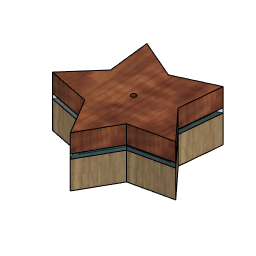
Star Prototype Non-Layered v3 (Autodesk Fusion 360 design; units mm, degrees)
Autodesk Fusion 360 part; units mm, degrees
note: some values were not read from the file. Set by a fixed rule: which face or edge a step refers to.
sketch "Sketch1" plane through (0, 0, 0) normal (0, 0, 1) x (1, 0, 0)
  line L0 (-201.2816, 81.9301) -> (-144.1352, 82.5743)
  line L1 (-144.1352, 82.5743) -> (-127.0887, 137.1228)
  line L2 (-127.0887, 137.1228) -> (-173.6998, 170.1914)
  line L3 (-173.6998, 170.1914) -> (-219.5535, 136.0805)
  line L4 (-219.5535, 136.0805) -> (-201.2816, 81.9301)
  line L5 (-196.6266, 153.136) -> (-226.1895, 192.8759) construction
  line L6 (-219.5535, 136.0805) -> (-226.1895, 192.8759)
  line L7 (-226.1895, 192.8759) -> (-173.6998, 170.1914)
  line L8 (-150.3942, 153.6571) -> (-121.7348, 194.0534) construction
  line L9 (-135.612, 109.8486) -> (-88.3366, 95.0749) construction
  line L10 (-172.7084, 82.2522) -> (-172.1501, 32.7254) construction
  line L11 (-210.4176, 109.0053) -> (-257.3479, 93.1697) construction
  line L12 (-173.6998, 170.1914) -> (-121.7348, 194.0534)
  line L13 (-127.0887, 137.1228) -> (-121.7348, 194.0534)
  line L14 (-127.0887, 137.1228) -> (-88.3366, 95.0749)
  line L15 (-144.1352, 82.5743) -> (-88.3366, 95.0749)
  line L16 (-144.1352, 82.5743) -> (-172.1501, 32.7254)
  line L17 (-257.3479, 93.1697) -> (-219.5535, 136.0805)
  circle A0 centre (-173.1518, 121.5798) radius 88.9 construction
  line L18 (-201.2816, 81.9301) -> (-257.3479, 93.1697)
  line L19 (-201.2816, 81.9301) -> (-172.1501, 32.7254)
  point P0 (-173.1518, 121.5798)
  dimension "d3" = 57.15
  dimension "d6" = 49.53
  dimension "d7" = 49.53
  dimension "d8" = 49.53
  dimension "d9" = 49.53
  dimension "d10" = 49.53
  dimension "d12" = 177.8
  constraint midpoint L3 L5.start
  constraint perpendicular L3 L5
  constraint midpoint L2 L8.start
  constraint perpendicular L2 L8
  constraint midpoint L1 L9.start
  constraint perpendicular L1 L9
  constraint midpoint L0 L10.start
  constraint perpendicular L0 L10
  constraint midpoint L4 L11.start
  constraint perpendicular L4 L11
  constraint coincident P0 A0.centre
  measures "d3" distance of L0.start L0.end
  measures "d6" distance of L5.start L5.end
  measures "d7" distance of L8.start L8.end
  measures "d8" distance of L9.start L9.end
  measures "d9" distance of L10.start L10.end
  measures "d10" distance of L11.start L11.end
  measures "d12" diameter of A0
extrude "Extrude1" add sketch "Sketch1" along normal blind 6.35 makes body 1
copy_body "CopyPasteBodies1" bodies 1 makes body 2
move_body "Move1" bodies 2 to x (1, 0, 0) y (0, 1, 0) z (0, 0, 1) at (0, 0, 6.35)
copy_body "CopyPasteBodies2" bodies 2 makes body 3
move_body "Move2" bodies 3 to x (1, 0, 0) y (0, 1, 0) z (0, 0, 1) at (0, 0, 6.35)
copy_body "CopyPasteBodies3" bodies 3 makes body 4
move_body "Move3" bodies 4 to x (1, 0, 0) y (0, 1, 0) z (0, 0, 1) at (0, 0, 6.35)
copy_body "CopyPasteBodies4" bodies 4 makes body 5
move_body "Move4" bodies 5 to x (1, 0, 0) y (0, 1, 0) z (0, 0, 1) at (0, 0, 6.35)
shell "Shell1" thickness 6.0325 removed faces 1 at (-163.5925, 118.5925, 31.75) on bodies 5
extrude "Extrude2" cut 1 faces at (-168.144, 128.6385, 31.4325) along direction (0, 0, -1) blind 6.0325 on bodies 5 bodies 5
copy_body "CopyPasteBodies6" bodies 5 makes body 6
move_body "Move5" bodies 6 to x (1, 0, 0) y (0, 1, 0) z (0, 0, 1) at (0, 0, 6.35)
copy_body "CopyPasteBodies7" bodies 6 makes body 7
move_body "Move6" bodies 7 to x (1, 0, 0) y (0, 1, 0) z (0, 0, 1) at (0, 0, 6.35)
copy_body "CopyPasteBodies8" bodies 1 2 3 4 makes body 8 makes body 9 makes body 10 makes body 11
move_body "Move7" bodies 8 9 10 11 to x (1, 0, 0) y (0, 1, 0) z (0, 0, 1) at (0, 0, 44.45)
sketch "Sketch2" plane through (0, 0, 69.85) normal (0, 0, 1) x (-1, 0, 0)
  line L0 (257.3479, -93.1697) -> (201.2816, -81.9301)
  line L1 (201.2816, -81.9301) -> (172.1501, -32.7254)
  line L2 (172.1501, -32.7254) -> (144.1352, -82.5743)
  line L3 (144.1352, -82.5743) -> (88.3366, -95.0749)
  line L4 (88.3366, -95.0749) -> (127.0887, -137.1228)
  line L5 (127.0887, -137.1228) -> (121.7348, -194.0534)
  line L6 (121.7348, -194.0534) -> (173.6998, -170.1914)
  line L7 (173.6998, -170.1914) -> (226.1895, -192.8759)
  line L8 (226.1895, -192.8759) -> (219.5535, -136.0805)
  line L9 (219.5535, -136.0805) -> (257.3479, -93.1697)
  line L10 (172.1501, -32.7254) -> (173.6998, -170.1914) construction
  line L11 (121.7348, -194.0534) -> (201.2816, -81.9301) construction
  line L12 (144.1352, -82.5743) -> (226.1895, -192.8759) construction
  circle A0 centre (173.1518, -121.5798) radius 3.175
  dimension "d20" = 6.35
  constraint coincident L1.end L2.start
  constraint coincident L6.end L7.start
  constraint coincident L5.end L6.start
  constraint coincident L0.end L1.start
  constraint coincident L2.end L3.start
  constraint coincident L7.end L8.start
  constraint coincident L10 A0.centre
  constraint coincident L12 A0.centre
  measures "d20" diameter of A0
extrude "Extrude3" cut sketch "Sketch2" against normal blind 25.4 contours A0 bodies 8 9 10 11
sketch "Sketch3" plane through (0, 0, 0) normal (0, 0, -1) x (1, 0, 0)
  line L0 (-201.2816, -81.9301) -> (-257.3479, -93.1697)
  line L1 (-257.3479, -93.1697) -> (-219.5535, -136.0805)
  line L2 (-219.5535, -136.0805) -> (-226.1895, -192.8759)
  line L3 (-226.1895, -192.8759) -> (-173.6998, -170.1914)
  line L4 (-173.6998, -170.1914) -> (-121.7348, -194.0534)
  line L5 (-121.7348, -194.0534) -> (-127.0887, -137.1228)
  line L6 (-127.0887, -137.1228) -> (-88.3366, -95.0749)
  line L7 (-88.3366, -95.0749) -> (-144.1352, -82.5743)
  line L8 (-144.1352, -82.5743) -> (-172.1501, -32.7254)
  line L9 (-172.1501, -32.7254) -> (-201.2816, -81.9301)
  line L10 (-226.1895, -192.8759) -> (-144.1352, -82.5743) construction
  line L11 (-201.2816, -81.9301) -> (-121.7348, -194.0534) construction
  line L12 (-172.1501, -32.7254) -> (-173.6998, -170.1914) construction
  circle A0 centre (-173.1518, -121.5798) radius 12.7
  dimension "d24" = 25.4
  constraint coincident L2.end L3.start
  constraint coincident L7.end L8.start
  constraint coincident L0.start L9.end
  constraint coincident L4.end L5.start
  constraint coincident L8.end L9.start
  constraint coincident L3.end L4.start
  constraint coincident L10 A0.centre
  constraint coincident L11 A0.centre
  measures "d24" diameter of A0
extrude "Extrude4" cut sketch "Sketch3" against normal blind 25.4 contours A0 bodies 1 2 3 4
combine "Combine1" operation add target body 1 tool bodies 4 2 3
combine "Combine2" operation add target body 8 tool bodies 11 10 9
combine "Combine3" operation add target body 5 tool bodies 6
combine "Combine4" operation add target body 5 tool bodies 1
equation "starInnerPolyEdgeLength = 2.25 in"
equation "d3 = starInnerPolyEdgeLength"
equation "starBranchLength = 1.95 in"
equation "d6 = starBranchLength"
equation "d7 = starBranchLength"
equation "d8 = starBranchLength"
equation "d9 = starBranchLength"
equation "d10 = starBranchLength"
equation "starOuterLayerThickness = 0.25 in"
equation "d13 = starOuterLayerThickness"
equation "d15 = starOuterLayerThickness * 0.95"
equation "d16 = -starOuterLayerThickness * 0.95"
equation "starLightEntranceDiameter = 0.25 in"
equation "d20 = starLightEntranceDiameter"
equation "d21 = -starOuterLayerThickness * 4"
equation "starRearMaintnenceInletDiameter = 1 in"
equation "d24 = starRearMaintnenceInletDiameter"
equation "d25 = -starOuterLayerThickness * 4"
named bodies: "layerBottom_1", "layerBottom_2", "layerBottom_3", "layerBottom_4", "layerInner_1", "layerInner_2", "layerInner_acrylic", "layerBottom_1 (1)", "layerBottom_2 (1)", "layerBottom_3 (1)", "layerBottom_4 (1)", "layerTop_1", "layerTop_2", "layerTop_3", "layerTop_4"
